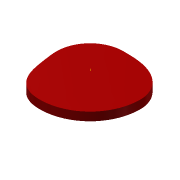
# Autodesk Inventor part: 凸輪
Saved by Autodesk Inventor 2015 SP2 (Build 190223200, 223)
## iProperties
Created: 2020-03-26
Part Number: 凸輪
Material: Stainless Steel, Austenitic
Document SubType Name: Modeling
Designer: Kuan-Lun Hsu
Manufacturer: Standard
Standards Organization: Custom
Density: 8 g/cm^3
Appearance: 平滑 - 紅色
Mass: 649.445 g
Surface Area: 195.848 cm^2
Volume: 81.1806 cm^3
CustomPartVersion: 1
Author: Kuan-Lun Hsu
Autodesk Inventor part; units mm, degrees
ref_plane "YZ Plane" through (0, 0, 0) normal (1, 0, 0) x (0, 1, 0)
ref_plane "XZ Plane" through (0, 0, 0) normal (0, 1, 0) x (-1, 0, 0)
ref_plane "XY Plane" through (0, 0, 0) normal (0, 0, 1) x (1, 0, 0)
sketch "主要草圖" plane through (0, 0, 0) normal (0, 0, 1) x (1, 0, 0)
  spline S0 degree 5 poles (0, 40) (1.152, 40.0133) (3.1519, 39.998) (6.3582, 39.9195) (10.2314, 39.8068) (15.4103, 39.4395) (20.2744, 38.8829) (25.4293, 37.9555) (30.5462, 36.6042) (35.6086, 34.7391) (40.5091, 32.2966) (45.1425, 29.2387) (49.3775, 25.5522) (53.0758, 21.2826) (56.1236, 16.4467) (58.3818, 11.2224) (59.8114, 5.5037) (60.1984, -0.0553) (59.7976, -6.4997) (58.8462, -12.5181) (57.2118, -18.6204) (54.9649, -24.4639) (52.1035, -30.0855) (48.6746, -35.3626) (44.711, -40.2586) (40.2582, -44.7109) (35.3638, -48.6744) (30.0827, -52.1042) (24.4705, -54.963) (18.5965, -57.2193) (12.5238, -58.8441) (6.3582, -59.8284) (0.1313, -60.1534) (-5.9667, -59.8732) (-11.7224, -58.8076) (-17.0697, -56.8839) (-21.8674, -54.0833) (-26.0258, -50.4647) (-29.4783, -46.1447) (-32.2131, -41.2869) (-34.2779, -36.0726) (-35.7853, -30.6718) (-36.8942, -25.2173) (-37.7767, -19.813) (-38.5595, -14.5315) (-39.2783, -9.4709) (-39.8428, -4.6435) (-40.1216, -0.1661) (-39.9003, 4.0983) (-39.2406, 8.3201) (-38.148, 12.3882) (-36.6423, 16.3151) (-34.7361, 20.0545) (-32.4494, 23.5762) (-29.8077, 26.8386) (-26.8379, 29.8076) (-23.5779, 32.4491) (-20.0505, 34.737) (-16.3244, 36.64) (-12.5289, 38.0912) (-8.5539, 39.1835) (-5.1078, 39.7534) (-2.7354, 39.9367) (-1.05, 39.9879) (0, 40) knots 0 0 0 0 0 0 0.019507 0.032547 0.048888 0.065312 0.081844 0.098499 0.115286 0.132197 0.149217 0.166323 0.183493 0.200704 0.21794 0.235365 0.252974 0.270763 0.28873 0.306875 0.325021 0.343167 0.361312 0.379458 0.397603 0.415749 0.433894 0.45204 0.470185 0.488331 0.50643 0.524395 0.542151 0.559656 0.5769 0.593945 0.610906 0.627877 0.644907 0.662002 0.679121 0.696197 0.713134 0.729815 0.746105 0.761949 0.77739 0.792502 0.807395 0.822211 0.837026 0.851842 0.866658 0.881474 0.89629 0.911105 0.925921 0.940737 0.955553 0.970368 0.982221 1 1 1 1 1 1
  point P0 (10.067, 39.766)
  point P1 (15.1278, 39.411)
  point P2 (20.2181, 38.8077)
  point P3 (25.3322, 37.8692)
  point P4 (30.4406, 36.5048)
  point P5 (35.4839, 34.6313)
  point P6 (40.3726, 32.1829)
  point P7 (44.9919, 29.1205)
  point P8 (49.2108, 25.4387)
  point P9 (52.8936, 21.1686)
  point P10 (55.9114, 16.3778)
  point P11 (58.1532, 11.1662)
  point P12 (59.5338, 5.6591)
  point P13 (60, 0)
  point P14 (59.6713, -6.2717)
  point P15 (58.6889, -12.4747)
  point P16 (57.0634, -18.541)
  point P17 (54.8127, -24.4042)
  point P18 (51.9615, -30)
  point P19 (48.541, -35.2671)
  point P20 (44.5887, -40.1478)
  point P21 (40.1478, -44.5887)
  point P22 (35.2671, -48.541)
  point P23 (30, -51.9615)
  point P24 (24.4042, -54.8127)
  point P25 (18.541, -57.0634)
  point P26 (12.4747, -58.6889)
  point P27 (6.2717, -59.6713)
  point P28 (0, -60)
  point P29 (-6.1113, -59.6506)
  point P30 (-11.8257, -58.5375)
  point P31 (-17.0628, -56.6053)
  point P32 (-21.7527, -53.8484)
  point P33 (-25.8373, -50.3039)
  point P34 (-29.2686, -46.0562)
  point P35 (-32.0239, -41.2436)
  point P36 (-34.1331, -36.0417)
  point P37 (-35.6934, -30.6253)
  point P38 (-36.8547, -25.134)
  point P39 (-37.7783, -19.6692)
  point P40 (-38.5803, -14.3239)
  point P41 (-39.2811, -9.2027)
  point P42 (-39.7987, -4.4042)
  point P43 (-40, 0)
  point P44 (-39.7809, 4.1811)
  point P45 (-39.1259, 8.3165)
  point P46 (-38.0423, 12.3607)
  point P47 (-36.5418, 16.2695)
  point P48 (-34.641, 20)
  point P49 (-32.3607, 23.5114)
  point P50 (-29.7258, 26.7652)
  point P51 (-26.7652, 29.7258)
  point P52 (-23.5114, 32.3607)
  point P53 (-20, 34.641)
  point P54 (-16.2695, 36.5418)
  point P55 (-12.3607, 38.0423)
  point P56 (-8.3165, 39.1259)
  point P57 (-4.1811, 39.7809)
  constraints: 60 other
extrude "凸輪" add sketch "主要草圖" along normal mid plane 10
sketch "草圖2" plane through (0, 0, -5) normal (0, 0, -1) x (-1, 0, 0)
  circle A0 centre (0, 0) radius 5
  dimension "d4" = 10
  constraints: 1 centre point, 1 coincident
  measures "d4" diameter of A0
extrude "擠出2" add sketch "草圖2" along normal blind 10
body "Solid1"
